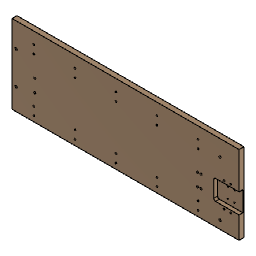
Y main board (Autodesk Fusion 360 design; units mm, degrees)
Autodesk Fusion 360 part; units mm, degrees
sketch "Front" plane through (0, 0, 0) normal (0, 1, 0) x (1, 0, 0)
  line L0 (415, -143.75) -> (-415, -143.75)
  line L1 (-415, -143.75) -> (-415, 143.75)
  line L2 (-415, 143.75) -> (415, 143.75)
  line L3 (415, 143.75) -> (415, -143.75)
  line L4 (415, -143.75) -> (-415, 143.75) construction
  line L5 (-415, -143.75) -> (415, 143.75) construction
  line L6 (-400, -101.125) -> (400, -101.125) construction
  line L7 (-400, -71.125) -> (400, -71.125) construction
  line L8 (-400, 93.875) -> (400, 93.875) construction
  line L9 (-400, 123.875) -> (400, 123.875) construction
  line L10 (-335, -110) -> (-335, 130) construction
  line L11 (-185, -110) -> (-185, 130) construction
  line L12 (-35, -110) -> (-35, 130) construction
  line L13 (115, -110) -> (115, 130) construction
  line L14 (265, -110) -> (265, 130) construction
  circle A0 centre (-335, -101.125) radius 3
  circle A1 centre (-335, -71.125) radius 3
  circle A2 centre (-335, 93.875) radius 3
  circle A3 centre (-335, 123.875) radius 3
  circle A4 centre (-185, 123.875) radius 3
  circle A5 centre (-185, 93.875) radius 3
  circle A6 centre (-185, -71.125) radius 3
  circle A7 centre (-185, -101.125) radius 3
  circle A8 centre (-35, -101.125) radius 3
  circle A9 centre (-35, -71.125) radius 3
  circle A10 centre (-35, 93.875) radius 3
  circle A11 centre (-35, 123.875) radius 3
  circle A12 centre (115, -101.125) radius 3
  circle A13 centre (115, -71.125) radius 3
  circle A14 centre (115, 93.875) radius 3
  circle A15 centre (115, 123.875) radius 3
  circle A16 centre (265, 123.875) radius 3
  circle A17 centre (265, 93.875) radius 3
  circle A18 centre (265, -71.125) radius 3
  circle A19 centre (265, -101.125) radius 3
  line L15 (-400, -120) -> (-400, 130) construction
  line L16 (345, -110) -> (345, 130) construction
  line L17 (-360, 49.875) -> (300, 49.875) construction
  line L18 (-360, 3.875) -> (300, 3.875) construction
  line L19 (-332, -10) -> (-332, 60) construction
  line L20 (263, -10) -> (263, 60) construction
  line L21 (276, -10) -> (276, 60) construction
  circle A20 centre (-332, 3.875) radius 3.5
  circle A21 centre (-332, 49.875) radius 3.5
  circle A22 centre (263, 3.875) radius 3.5
  circle A23 centre (276, 3.875) radius 3.5
  circle A24 centre (263, 49.875) radius 3.5
  circle A25 centre (276, 49.875) radius 3.5
  circle A26 centre (-400, -55) radius 4
  circle A27 centre (-400, 65) radius 4
  circle A28 centre (345, 114.875) radius 4
  circle A29 centre (345, -85.125) radius 4
  line L22 (415, -9.625) -> (322.5, -9.625)
  line L23 (322.5, -9.625) -> (322.5, 63.375)
  line L24 (322.5, 63.375) -> (415, 63.375)
  line L25 (415, 63.375) -> (415, -9.625)
  line L26 (384.5, -50) -> (384.5, 85) construction
  line L27 (360.5, -50) -> (360.5, 85) construction
  line L28 (355, -18.125) -> (390, -18.125) construction
  line L29 (350, 6.875) -> (390, 6.875) construction
  line L30 (350, 46.875) -> (390, 46.875) construction
  line L31 (350, 71.875) -> (390, 71.875) construction
  circle A30 centre (360.5, -18.125) radius 3
  circle A31 centre (384.5, -18.125) radius 3
  circle A32 centre (360.5, 71.875) radius 3
  circle A33 centre (384.5, 71.875) radius 3
  circle A34 centre (360.5, 46.875) radius 2.5
  circle A35 centre (384.5, 46.875) radius 2.5
  circle A36 centre (360.5, 6.875) radius 2.5
  circle A37 centre (384.5, 6.875) radius 2.5
  dimension "d1" = 830
  dimension "d2" = 287.5
  dimension "d3" = 30
  dimension "d4" = 30
  dimension "d5" = 165
  dimension "d6" = 19.875
  dimension "d7" = 150
  dimension "d8" = 150
  dimension "d9" = 150
  dimension "d10" = 150
  dimension "d11" = 80
  dimension "d12" = 6
  dimension "d13" = 6
  dimension "d14" = 6
  dimension "d15" = 6
  dimension "d16" = 6
  dimension "d17" = 6
  dimension "d18" = 6
  dimension "d19" = 6
  dimension "d20" = 6
  dimension "d21" = 6
  dimension "d22" = 6
  dimension "d23" = 6
  dimension "d24" = 6
  dimension "d25" = 6
  dimension "d26" = 6
  dimension "d27" = 6
  dimension "d28" = 6
  dimension "d29" = 6
  dimension "d30" = 6
  dimension "d31" = 6
  dimension "d32" = 15
  dimension "d33" = 70
  dimension "d34" = 46
  dimension "d36" = 75
  dimension "d37" = 83
  dimension "d38" = 13
  dimension "d39" = 595
  dimension "d40" = 7
  dimension "d41" = 7
  dimension "d42" = 7
  dimension "d43" = 7
  dimension "d44" = 7
  dimension "d45" = 7
  dimension "d46" = 8
  dimension "d47" = 8
  dimension "d48" = 120
  dimension "d49" = 78.75
  dimension "d50" = 8
  dimension "d51" = 8
  dimension "d52" = 200
  dimension "d54" = 16
  dimension "d55" = 745
  dimension "d56" = 92.5
  dimension "d57" = 73
  dimension "d58" = 13.5
  dimension "d59" = 24
  dimension "d60" = 30.5
  dimension "d61" = 25
  dimension "d62" = 25
  dimension "d63" = 40
  dimension "d64" = 16.5
  dimension "d65" = 6
  dimension "d66" = 6
  dimension "d67" = 6
  dimension "d68" = 6
  dimension "d69" = 5
  dimension "d70" = 5
  dimension "d71" = 5
  dimension "d72" = 5
  constraint perpendicular L0 L1
  constraint parallel L0 L2
  constraint parallel L1 L3
  constraint horizontal L0
  constraint coincident L4 origin
  constraint coincident L5 origin
  constraint parallel L0 L6
  constraint horizontal L7
  constraint horizontal L8
  constraint perpendicular L1 L9
  constraint perpendicular L9 L10
  constraint perpendicular L9 L11
  constraint perpendicular L9 L12
  constraint perpendicular L9 L13
  constraint perpendicular L9 L14
  constraint coincident L10 A0.centre
  constraint coincident L6 A0.centre
  constraint coincident L10 A1.centre
  constraint coincident L7 A1.centre
  constraint coincident L8 A2.centre
  constraint coincident L10 A2.centre
  constraint coincident L9 A3.centre
  constraint coincident L10 A3.centre
  constraint coincident L9 A4.centre
  constraint coincident L11 A4.centre
  constraint coincident L11 A5.centre
  constraint coincident L8 A5.centre
  constraint coincident L11 A6.centre
  constraint coincident L7 A6.centre
  constraint coincident L11 A7.centre
  constraint coincident L6 A7.centre
  constraint coincident L6 A8.centre
  constraint coincident L12 A8.centre
  constraint coincident L7 A9.centre
  constraint coincident L12 A9.centre
  constraint coincident L12 A10.centre
  constraint coincident L8 A10.centre
  constraint coincident L9 A11.centre
  constraint coincident L12 A11.centre
  constraint coincident L6 A12.centre
  constraint coincident L13 A12.centre
  constraint coincident L7 A13.centre
  constraint coincident L13 A13.centre
  constraint coincident L8 A14.centre
  constraint coincident L13 A14.centre
  constraint coincident L13 A15.centre
  constraint coincident L9 A15.centre
  constraint coincident L9 A16.centre
  constraint coincident L14 A16.centre
  constraint coincident L8 A17.centre
  constraint coincident L14 A17.centre
  constraint coincident L7 A18.centre
  constraint coincident L14 A18.centre
  constraint coincident L14 A19.centre
  constraint coincident L6 A19.centre
  constraint parallel L1 L15
  constraint perpendicular L9 L16
  constraint perpendicular L12 L17
  constraint perpendicular L14 L18
  constraint perpendicular L17 L19
  constraint perpendicular L17 L20
  constraint perpendicular L17 L21
  constraint coincident L18 A20.centre
  constraint coincident L19 A20.centre
  constraint coincident L17 A21.centre
  constraint coincident L19 A21.centre
  constraint coincident L18 A22.centre
  constraint coincident L20 A22.centre
  constraint coincident L21 A23.centre
  constraint coincident L18 A23.centre
  constraint coincident L17 A24.centre
  constraint coincident L20 A24.centre
  constraint coincident L21 A25.centre
  constraint coincident L17 A25.centre
  constraint coincident L15 A26.centre
  constraint coincident L15 A27.centre
  constraint coincident L16 A28.centre
  constraint coincident L16 A29.centre
  constraint horizontal L22
  constraint vertical L23
  constraint horizontal L24
  constraint vertical L25
  constraint coincident L3 L22.start
  constraint perpendicular L24 L26
  constraint perpendicular L22 L27
  constraint perpendicular L26 L28
  constraint perpendicular L26 L29
  constraint perpendicular L26 L30
  constraint perpendicular L26 L31
  constraint coincident L27 A30.centre
  constraint coincident L28 A30.centre
  constraint coincident L28 A31.centre
  constraint coincident L26 A31.centre
  constraint coincident L27 A32.centre
  constraint coincident L31 A32.centre
  constraint coincident L26 A33.centre
  constraint coincident L31 A33.centre
  constraint coincident L27 A34.centre
  constraint coincident L30 A34.centre
  constraint coincident L30 A35.centre
  constraint coincident L26 A35.centre
  constraint coincident L27 A36.centre
  constraint coincident L29 A36.centre
  constraint coincident L26 A37.centre
  constraint coincident L29 A37.centre
  measures "d1" distance of L1.end L2.end
  measures "d2" distance of L0.end L1.end
  measures "d3" distance of L6 L7
  measures "d4" distance of L8 L9
  measures "d5" distance of L7 L8
  measures "d6" distance of L2 L9
  measures "d7" distance of L13 L14
  measures "d8" distance of L12 L13
  measures "d9" distance of L11 L12
  measures "d10" distance of L10 L11
  measures "d11" distance of L1 L10
  measures "d12" diameter of A0
  measures "d13" diameter of A1
  measures "d14" diameter of A2
  measures "d15" diameter of A3
  measures "d16" diameter of A4
  measures "d17" diameter of A5
  measures "d18" diameter of A6
  measures "d19" diameter of A7
  measures "d20" diameter of A8
  measures "d21" diameter of A9
  measures "d22" diameter of A10
  measures "d23" diameter of A11
  measures "d24" diameter of A12
  measures "d25" diameter of A13
  measures "d26" diameter of A14
  measures "d27" diameter of A15
  measures "d28" diameter of A16
  measures "d29" diameter of A17
  measures "d30" diameter of A18
  measures "d31" diameter of A19
  measures "d32" distance of L1 L15
  measures "d33" distance of L3 L16
  measures "d34" distance of L17 L18
  measures "d36" distance of L7 L18
  measures "d37" distance of L1 L19
  measures "d38" distance of L20 L21
  measures "d39" distance of L19 L20
  measures "d40" diameter of A20
  measures "d41" diameter of A21
  measures "d42" diameter of A22
  measures "d43" diameter of A23
  measures "d44" diameter of A24
  measures "d45" diameter of A25
  measures "d46" diameter of A26
  measures "d47" diameter of A27
  measures "d48" distance of A26.centre A27.centre
  measures "d49" distance of L2 A27.centre
  measures "d50" diameter of A28
  measures "d51" diameter of A29
  measures "d52" distance of A28.centre A29.centre
  measures "d54" distance of L6 A29.centre
  measures "d55" distance of L15 L16
  measures "d56" distance of L22.start L22.end
  measures "d57" distance of L22.start L24.end
  measures "d58" distance of A23.centre L22
  measures "d59" distance of L26 L27
  measures "d60" distance of L3 L26
  measures "d61" distance of L30.end L31
  measures "d62" distance of L28 L29
  measures "d63" distance of L29 L30
  measures "d64" distance of L24 L30
  measures "d65" diameter of A30
  measures "d66" diameter of A31
  measures "d67" diameter of A32
  measures "d68" diameter of A33
  measures "d69" diameter of A34
  measures "d70" diameter of A35
  measures "d71" diameter of A36
  measures "d72" diameter of A37
extrude "Extrude1" add sketch "Front" against normal blind 4 contours L3 L22 L23 L24 L25
extrude "Extrude2" add sketch "Front" against normal blind 18 contours L0 L1 L2 L3 L22 L23 L24
fillet "Fillet1" radius 6.35 2 edges at (322.5, -11, -63.375) (322.5, -11, 9.625)
named bodies: "Y main board"
